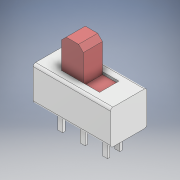
# Autodesk Inventor part: switch
Saved by Autodesk Inventor 2020 (Build 240168000, 168)
## iProperties
Created: 2020-11-29
Part Number: switch
Material: PAEK Plastic
Document SubType Name: Modeling
Designer: Milosz
Density: 1.32 g/cm^3
Appearance: Smooth - White
Author: Milosz
Autodesk Inventor part; units mm, degrees
ref_plane "YZ Plane" through (0, 0, 0) normal (1, 0, 0) x (0, 1, 0)
ref_plane "XZ Plane" through (0, 0, 0) normal (0, 1, 0) x (-1, 0, 0)
ref_plane "XY Plane" through (0, 0, 0) normal (0, 0, 1) x (1, 0, 0)
sketch "Sketch1" plane through (0, 0, 0) normal (0, 1, 0) x (-1, 0, 0)
  line L0 (17.8833, -8.321) -> (1.6833, -8.321)
  line L1 (1.6833, -8.321) -> (1.6833, -0.721)
  line L2 (1.6833, -0.721) -> (17.8833, -0.721)
  line L3 (17.8833, -0.721) -> (17.8833, -8.321)
  dimension "d23" = 16.2
  constraints: 8 end point, 2 parallel, 1 horizontal, 1 perpendicular
  measures "d23" distance of L1.end L2.end
extrude "Extrusion5" add sketch "Sketch1" along normal blind 7.2
fillet "Fillet2" radius 0.5 4 edges at (-9.7833, 7.2, -0.721) (-9.7833, 7.2, -8.321) (-9.7833, 0, -0.721) (-9.7833, 0, -8.321)
sketch "Sketch7" plane through (0, 7.2, 0) normal (0, 1, 0) x (1, 0, 0)
  line L0 (-17.8833, 7.821) -> (-1.6833, 7.821) projected
  line L1 (-17.8833, 7.821) -> (-17.8833, 1.221) projected
  line L2 (-1.6833, 1.221) -> (-17.8833, 1.221) projected
  line L3 (-1.6833, 1.221) -> (-1.6833, 7.821) projected
  line L4 (-13.8133, 2.491) -> (-5.7533, 2.491)
  line L5 (-5.7533, 2.491) -> (-5.7533, 6.551)
  line L6 (-5.7533, 6.551) -> (-13.8133, 6.551)
  line L7 (-13.8133, 6.551) -> (-13.8133, 2.491)
  line L8 (-13.8133, 2.491) -> (-5.7533, 6.551) construction
  line L9 (-5.7533, 2.491) -> (-13.8133, 6.551) construction
  point P0 (0, 0)
  point P1 (-9.7833, 4.521)
  dimension "d28" = 8.06
  dimension "d29" = 4.06
  constraints: 12 end point, 2 midpoint, 2 parallel, 1 horizontal, 1 perpendicular
  measures "d28" distance of L6.end L5.end
  measures "d29" distance of L5.end L4.end
extrude "Extrusion6" cut sketch "Sketch7" against normal blind 0.5 contours L7 L6 L5 L4
sketch "Sketch8" plane through (0, 6.7, 0) normal (0, 1, 0) x (1, 0, 0)
  line L0 (-13.7727, 6.521) -> (-9.1727, 6.521)
  line L1 (-9.1727, 6.521) -> (-9.1727, 2.521)
  line L2 (-9.1727, 2.521) -> (-13.7727, 2.521)
  line L3 (-13.7727, 2.521) -> (-13.7727, 6.521)
  line L4 (-13.7727, 6.521) -> (-9.1727, 2.521) construction
  line L5 (-9.1727, 6.521) -> (-13.7727, 2.521) construction
  line L6 (-13.8133, 6.551) -> (-5.7533, 6.551) projected
  line L7 (-13.8133, 2.491) -> (-13.8133, 6.551) projected
  line L8 (-5.7533, 2.491) -> (-13.8133, 2.491) projected
  line L9 (-5.7533, 6.551) -> (-5.7533, 2.491) projected
  point P0 (0, 0)
  point P1 (-11.4727, 4.521)
  dimension "d32" = 4.6
  dimension "d33" = 4
  dimension "d34" = 2.03
  constraints: 12 end point, 2 midpoint, 2 parallel, 1 horizontal, 1 perpendicular
  measures "d32" distance of L1.end L2.end
  measures "d33" distance of L0.end L1.end
  measures "d34" distance from line of L6 point (-11.473, 4.521)
extrude "Extrusion7" add sketch "Sketch8" along normal blind 7 contours L0 L1 L2 L3
chamfer "Chamfer1" distance 1 angle 45 2 edges at (-9.1727, 13.7, -4.521) (-13.7727, 13.7, -4.521)
sketch "Sketch9" plane through (0, 0, 0) normal (0, -1, 0) x (1, 0, 0)
  line L0 (-1.6833, -7.821) -> (-17.8833, -7.821) projected
  line L1 (-1.6833, -1.221) -> (-1.6833, -7.821) projected
  line L2 (-17.8833, -1.221) -> (-1.6833, -1.221) projected
  line L3 (-17.8833, -7.821) -> (-17.8833, -1.221) projected
  line L4 (-5.5833, -2.991) -> (-4.5833, -2.991)
  line L5 (-4.5833, -2.991) -> (-4.5833, -3.491)
  line L6 (-4.5833, -3.491) -> (-5.5833, -3.491)
  line L7 (-5.5833, -3.491) -> (-5.5833, -2.991)
  line L8 (-5.5833, -2.991) -> (-4.5833, -3.491) construction
  line L9 (-4.5833, -2.991) -> (-5.5833, -3.491) construction
  line L10 (-10.2833, -2.991) -> (-9.2833, -2.991)
  line L11 (-9.2833, -2.991) -> (-9.2833, -3.491)
  line L12 (-9.2833, -3.491) -> (-10.2833, -3.491)
  line L13 (-10.2833, -3.491) -> (-10.2833, -2.991)
  line L14 (-10.2833, -2.991) -> (-9.2833, -3.491) construction
  line L15 (-9.2833, -2.991) -> (-10.2833, -3.491) construction
  line L16 (-14.9833, -2.991) -> (-13.9833, -2.991)
  line L17 (-13.9833, -2.991) -> (-13.9833, -3.491)
  line L18 (-13.9833, -3.491) -> (-14.9833, -3.491)
  line L19 (-14.9833, -3.491) -> (-14.9833, -2.991)
  line L20 (-14.9833, -2.991) -> (-13.9833, -3.491) construction
  line L21 (-13.9833, -2.991) -> (-14.9833, -3.491) construction
  line L22 (-5.5833, -5.551) -> (-4.5833, -5.551)
  line L23 (-4.5833, -5.551) -> (-4.5833, -6.051)
  line L24 (-4.5833, -6.051) -> (-5.5833, -6.051)
  line L25 (-5.5833, -6.051) -> (-5.5833, -5.551)
  line L26 (-5.5833, -5.551) -> (-4.5833, -6.051) construction
  line L27 (-4.5833, -5.551) -> (-5.5833, -6.051) construction
  line L28 (-10.2833, -5.551) -> (-9.2833, -5.551)
  line L29 (-9.2833, -5.551) -> (-9.2833, -6.051)
  line L30 (-9.2833, -6.051) -> (-10.2833, -6.051)
  line L31 (-10.2833, -6.051) -> (-10.2833, -5.551)
  line L32 (-10.2833, -5.551) -> (-9.2833, -6.051) construction
  line L33 (-9.2833, -5.551) -> (-10.2833, -6.051) construction
  line L34 (-14.9833, -5.551) -> (-13.9833, -5.551)
  line L35 (-13.9833, -5.551) -> (-13.9833, -6.051)
  line L36 (-13.9833, -6.051) -> (-14.9833, -6.051)
  line L37 (-14.9833, -6.051) -> (-14.9833, -5.551)
  line L38 (-14.9833, -5.551) -> (-13.9833, -6.051) construction
  line L39 (-13.9833, -5.551) -> (-14.9833, -6.051) construction
  line L40 (-1.6833, -1.221) -> (-17.8833, -1.221) projected
  line L41 (-9.7833, -1.221) -> (-9.7833, -7.821) construction
  line L42 (-17.8833, -7.821) -> (-1.6833, -7.821) projected
  line L43 (-1.6833, -1.221) -> (-1.6833, -7.821) projected
  line L44 (-1.6833, -4.521) -> (-17.8833, -4.521) construction
  line L45 (-17.8833, -7.821) -> (-17.8833, -1.221) projected
  point P0 (0, 0)
  point P1 (-5.0833, -3.241)
  point P2 (-9.7833, -3.241)
  point P3 (-14.4833, -3.241)
  point P4 (-5.0833, -5.801)
  point P5 (-9.7833, -5.801)
  point P6 (-14.4833, -5.801)
  point P7 (-9.7833, -3.241)
  dimension "d40" = 1
  dimension "d41" = 0.5
  dimension "d44" = 4.7
  dimension "d47" = 2.56
  dimension "d50" = 1.28
  constraints: 76 end point, 17 midpoint, 2 horizontal, 2 parallel, 1 perpendicular, 1 point on line, 1 vertical, 55 other
  measures "d40" distance of L5.end L6.end
  measures "d41" distance of L4.end L5.end
  measures "d44" distance of L4.start L10.start
  measures "d47" distance of L4.start L22.start
  measures "d50" distance from line of point (-9.783, -3.241) L44
extrude "Extrusion8" add sketch "Sketch9" along normal blind 4.5 contours L4 L5 L6 L7 | L10 L11 L12 L13 | L16 L17 L18 L19 | L22 L23 L24 L25 | L28 L29 L30 L31 | L34 L35 L36 L37
equation "\"d34\" = 0.5 * d29"
equation "\"d50\" = 0.5 * d47"
body "Solid2"
